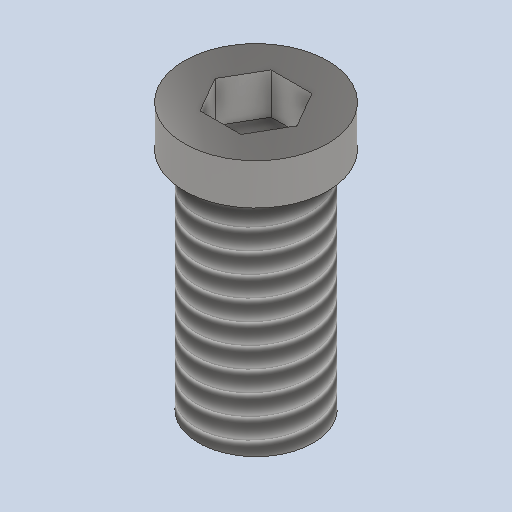
# Autodesk Inventor part: Connector_3
Saved by Autodesk Inventor 2022 (Build 260153000, 153)
## iProperties
Created: 2023-01-17
Part Number: Connector_3
Material: Steel, Mild
Document SubType Name: Modeling
Designer: 48735
Density: 7.85 g/cm^3
Appearance: Semi-Polished
Author: 48735
Autodesk Inventor part; units mm, degrees
ref_plane "YZ Plane" through (0, 0, 0) normal (1, 0, 0) x (0, 1, 0)
ref_plane "XZ Plane" through (0, 0, 0) normal (0, 1, 0) x (-1, 0, 0)
ref_plane "XY Plane" through (0, 0, 0) normal (0, 0, 1) x (1, 0, 0)
sketch "Sketch1" plane through (0, 0, 0) normal (0, 1, 0) x (-1, 0, 0)
  circle A0 centre (0, 0) radius 1.4
  dimension "d0" = 2.8
  constraints: 1 centre point, 1 coincident
  measures "d0" diameter of A0
extrude "Extrusion1" add sketch "Sketch1" along normal blind 5.5
sketch "Sketch2" plane through (0, 5.5, 0) normal (0, 1, 0) x (1, 0, 0)
  circle A0 centre (0, 0) radius 1.75
  line L0 (0, 0) -> (-1, 0)
  line L1 (-1, 0) -> (-0.5, 0.866)
  line L2 (-0.5, 0.866) -> (0.5, 0.866)
  line L3 (0.5, 0.866) -> (1, 0)
  line L4 (1, 0) -> (0.5, -0.866)
  line L5 (0.5, -0.866) -> (-0.5, -0.866)
  line L6 (-0.5, -0.866) -> (-1, 0)
  dimension "d3" = 3.5
  dimension "d4" = 1
  constraints: 14 end point, 2 coincident, 1 centre point, 1 horizontal, 13 other
  measures "d3" diameter of A0
  measures "d4" distance of L0.start L0.end
extrude "Extrusion2" add sketch "Sketch2" along normal blind 1
thread "Thread1" size "M3x0.5" class "6g" standard "ANSI Metric M Profile" length 6
body "Solid1"
